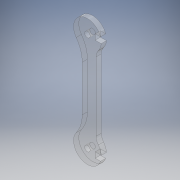
# Autodesk Inventor part: Spacer2
Saved by Autodesk Inventor 2017 (Build 210142000, 142)
## iProperties
Created: 2017-04-16
Part Number: Spacer2
Material: Generic
Document SubType Name: Modeling
Designer: jeffkub
Density: 1 g/cm^3
Appearance: Polycarbonate - Clear
Author: jeffkub
Autodesk Inventor part; units mm, degrees
ref_plane "YZ Plane" through (0, 0, 0) normal (1, 0, 0) x (0, 1, 0)
ref_plane "XZ Plane" through (0, 0, 0) normal (0, 1, 0) x (-1, 0, 0)
ref_plane "XY Plane" through (0, 0, 0) normal (0, 0, 1) x (1, 0, 0)
sketch "Sketch2" plane through (0, 0, 0) normal (0, 1, 0) x (-1, 0, 0)
  line L0 (3, -13.1703) -> (3, 0)
  line L1 (-7.9775, -27.9) -> (-4.5, -27.9)
  line L2 (-4.5, -27.9) -> (-4.5, -31.1)
  line L3 (-4.5, -31.1) -> (-7.5657, -31.1)
  circle A0 centre (0, -28.5) radius 1.6
  line L4 (-5, -19.8397) -> (-5, 0)
  arc A1 (-6.2857, -23.5513) -> (-7.9775, -27.9) centre (0, -28.5) ccw
  arc A2 (-7.5657, -31.1) -> (6.4615, -23.7832) centre (0, -28.5) ccw
  line L5 (62.6119, 0) -> (-52.77, 0)
  arc A3 (3, -13.1703) -> (6.4615, -23.7832) centre (21, -13.1703) ccw
  line L6 (3, 0) -> (-5, 0)
  arc A4 (-6.2857, -23.5513) -> (-5, -19.8397) centre (-11, -19.8397) ccw
  point P0 (0, 0)
  point P1 (0, 0)
  point P2 (-5, -22.255)
  point P3 (3, -21.0838)
  dimension "d3" = 0.6
  dimension "d4" = 3.2
  dimension "d5" = 3.2
  dimension "d6" = 4.5
  dimension "d8" = 57
  dimension "d9" = 3
  dimension "d10" = 5
  dimension "d11" = 8
  dimension "d12" = 18
  dimension "d15" = 6
  constraints: 14 end point, 10 point on circle, 5 centre point, 5 point on line, 4 tangent, 3 horizontal, 2 coincident, 2 vertical, 1 collinear, 1 concentric, 1 perpendicular, 1 vertical alignment
  measures "d3" distance from line of L1 A1.centre
  measures "d4" distance between parallel lines of L1 L3
  measures "d5" diameter of A0
  measures "d6" distance from line of L2 A1.centre
  measures "d8" diameter of A1.centre L5
  measures "d9" distance from line of point (0, 0) L0
  measures "d10" distance from line of point (0, 0) L4
  measures "d11" radius of A2
  measures "d12" radius of A3
  measures "d15" radius of A4
extrude "Extrusion1" add sketch "Sketch2" along normal blind 3
mirror "Mirror1" about plane through (0, 0, 0) normal (0, 0, 1) of "Extrusion1"
body "Solid1"
